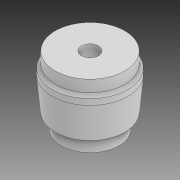
# Autodesk Inventor part: Cablecar_spacer
Saved by Autodesk Inventor 2020 (Build 240168000, 168)
## iProperties
Created: 2021-02-03
Part Number: Cablecar_spacer
Material: Generic
Document SubType Name: Modeling
Designer: DDeGo
Density: 1 g/cm^3
Appearance: Default
Author: DDeGo
Autodesk Inventor part; units mm, degrees
ref_plane "YZ Plane" through (0, 0, 0) normal (1, 0, 0) x (0, 1, 0)
ref_plane "XZ Plane" through (0, 0, 0) normal (0, 1, 0) x (-1, 0, 0)
ref_plane "XY Plane" through (0, 0, 0) normal (0, 0, 1) x (1, 0, 0)
sketch "Sketch1" plane through (0, 0, 0) normal (0, 0, 1) x (1, 0, 0)
  line L0 (1.45, -3.5) -> (1.45, 0.5) construction
  line L1 (1.45, 3.5) -> (5.9, 3.5) construction
  line L2 (6.4, 3) -> (6.4, 2)
  line L3 (4.9, -3.5) -> (3, -3.5) construction
  line L4 (0, 0) -> (0, 3.5) construction
  line L5 (0, 3.5) -> (1.45, 3.5) construction
  line L6 (0, 0) -> (0, -3.5) construction
  line L7 (0, -3.5) -> (1.45, -3.5) construction
  line L8 (1.45, 3.5) -> (1.45, 5.5)
  line L9 (1.45, 5.5) -> (5.9, 5.5)
  line L10 (5.9, 5.5) -> (5.9, 3.5)
  line L11 (5.9, 3.5) -> (6.4, 3)
  line L12 (3, -3.5) -> (3, 0.5)
  line L13 (3, 0.5) -> (1.45, 0.5)
  line L14 (1.45, 0.5) -> (1.45, 3.5)
  line L15 (3, -3.5) -> (1.45, -3.5) construction
  line L16 (3, -3.5) -> (3, -6)
  line L17 (3, -6) -> (4.9, -6)
  line L18 (4.9, -6) -> (4.9, -3.5)
  line L19 (4.9, -3.5) -> (5.9, -3.5)
  line L20 (5.9, -3.5) -> (6.4, 2)
  dimension "d0" = 7
  dimension "d1" = 1.45
  dimension "d2" = 5.9
  dimension "d4" = 2
  dimension "d5" = 3
  dimension "d6" = 5
  dimension "d7" = 135
  dimension "d8" = 0.5
  dimension "d12" = 2.5
  dimension "d13" = 4.9
  dimension "d14" = 1
  dimension "d15" = 1
  constraints: 42 end point, 14 perpendicular, 3 vertical, 2 parallel, 1 collinear, 1 horizontal, 1 point on line
  measures "d0" distance between parallel lines of L3 L1
  measures "d1" distance between parallel lines of L4 L0
  measures "d2" distance between parallel lines of L4 L10
  measures "d4" distance of L9.end L1.end
  measures "d5" distance between parallel lines of L6 L12
  measures "d6" distance between parallel lines of L9 L13
  measures "d7" angle of L11 L10
  measures "d8" distance between parallel lines of L2 L10
  measures "d12" distance of L17.end L3.start
  measures "d13" distance between parallel lines of L6 L18
  measures "d14" distance of L3.start L19.end
  measures "d15" distance of L2.start L2.end
revolve "Revolution1" add sketch "Sketch1" angle 360 about axis through (0, 0, 0) along (0, 1, 0)
body "Solid1"
